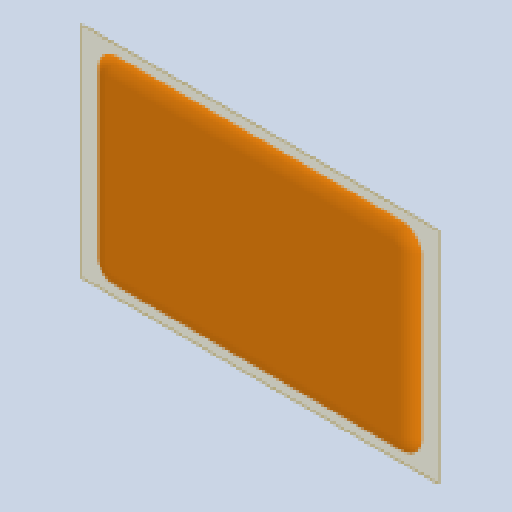
# Autodesk Inventor part: крышка головы
Saved by Autodesk Inventor 2024.2 (Build 282272000, 272)
## iProperties
Created: 2025-10-19
Part Number: крышка головы
Material: Типовые
Document SubType Name: Modeling
Designer: katya_notebook
Density: 1 g/cm^3
Appearance: Оранжевый
Author: katya_notebook
Autodesk Inventor part; units mm, degrees
ref_plane "YZ Plane" through (0, 0, 0) normal (1, 0, 0) x (0, 1, 0)
ref_plane "XZ Plane" through (0, 0, 0) normal (0, 1, 0) x (-1, 0, 0)
ref_plane "XY Plane" through (0, 0, 0) normal (0, 0, 1) x (1, 0, 0)
ref_plane "РабПлоскость1" through (0, 0, 0) normal (0, 0, 1) x (1, 0, 0)
sketch "Эскиз1" plane through (0, 0, 0) normal (0, 0, 1) x (1, 0, 0)
  arc A0 (65, 32) -> (57, 40) centre (57, 32) ccw projected
  line L0 (65, -32) -> (65, 32) projected
  line L1 (57, 40) -> (-57, 40) projected
  arc A1 (-57, 40) -> (-65, 32) centre (-57, 32) ccw projected
  line L2 (-65, 32) -> (-65, -32) projected
  arc A2 (-65, -32) -> (-57, -40) centre (-57, -32) ccw projected
  line L3 (-57, -40) -> (57, -40) projected
  arc A3 (57, -40) -> (65, -32) centre (57, -32) ccw projected
  line L4 (65, 32) -> (65, -32)
  line L5 (57, -40) -> (-57, -40)
  line L6 (-65, -32) -> (-65, 32)
  line L7 (-57, 40) -> (57, 40)
  arc A4 (65, 32) -> (57, 40) centre (57, 32) ccw
  arc A5 (57, -40) -> (65, -32) centre (57, -32) ccw
  arc A6 (-65, -32) -> (-57, -40) centre (-57, -32) ccw
  arc A7 (-57, 40) -> (-65, 32) centre (-57, 32) ccw
  point P0 (0, 0)
  constraints: 8 end point, 8 point on circle, 6 tangent, 4 centre point, 3 collinear, 1 concentric, 1 perpendicular
extrude "Выдавливание1" add sketch "Эскиз1" along normal blind 3
fillet "Сопряжение1" radius 8 8 edges at (-62.6569, 37.6569, 3) (-65, 0, 3) (-62.6569, -37.6569, 3) (0, -40, 3) (62.6569, -37.6569, 3) (65, 0, 3) (62.6569, 37.6569, 3) (0, 40, 3)
